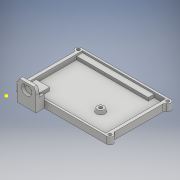
# Autodesk Inventor part: Redid DAQ Enclosure Bottom TTL
Saved by Autodesk Inventor 2017 (Build 210142000, 142)
## iProperties
Created: 2017-07-24
Part Number: Redid DAQ Enclosure Bottom TTL
Material: Generic
Document SubType Name: Modeling
Designer: andrew
Density: 1 g/cm^3
Appearance: Default
Author: andrew
Autodesk Inventor part; units mm, degrees
ref_plane "YZ Plane" through (0, 0, 0) normal (1, 0, 0) x (0, 1, 0)
ref_plane "XZ Plane" through (0, 0, 0) normal (0, 1, 0) x (-1, 0, 0)
ref_plane "XY Plane" through (0, 0, 0) normal (0, 0, 1) x (1, 0, 0)
sketch "Sketch1" plane through (0, 0, 0) normal (0, 0, 1) x (1, 0, 0)
  line L0 (85.72, 30.226) -> (85.72, 1.401) construction
  line L1 (85.72, 1.401) -> (45.72, 1.401) construction
  line L2 (85.72, 1.401) -> (5.72, 1.401) construction
  line L3 (5.72, 1.401) -> (5.72, 59.001) construction
  line L4 (5.72, 59.001) -> (85.72, 59.001) construction
  line L5 (85.72, 59.001) -> (85.72, 1.401) construction
  line L6 (61.99, 1.401) -> (61.99, 20.221) construction
  line L7 (61.99, 20.221) -> (85.72, 20.221) construction
  line L8 (61.99, 20.221) -> (58.44, 20.221) construction
  line L9 (61.99, 23.771) -> (61.99, 20.221) construction
  line L10 (60.215, 20.221) -> (61.99, 20.221) construction
  line L11 (61.99, 20.221) -> (61.99, 21.996) construction
  line L12 (61.99, 21.996) -> (60.215, 21.996) construction
  line L13 (60.215, 21.996) -> (60.215, 20.221) construction
  circle A0 centre (60.215, 21.996) radius 1.775 construction
  circle A1 centre (60.215, 21.996) radius 2.775 construction
  circle A2 centre (60.215, 21.996) radius 4.275 construction
  line L14 (5.72, 59.001) -> (74.72, 59.001) construction
  line L15 (74.72, 59.001) -> (74.72, 53.301) construction
  line L16 (74.72, 53.301) -> (5.72, 53.301) construction
  line L17 (5.72, 53.301) -> (5.72, 59.001) construction
  line L18 (5.72, 1.401) -> (18.72, 1.401) construction
  line L19 (18.72, 1.401) -> (18.72, 14.401) construction
  line L20 (18.72, 14.401) -> (5.72, 14.401) construction
  line L21 (5.72, 14.401) -> (5.72, 1.401) construction
  circle A3 centre (2.72, 58.001) radius 1.5
  line L22 (3.72, 61.001) -> (5.72, 61.001)
  line L23 (5.72, 61.001) -> (5.72, 59.001) construction
  line L24 (5.72, 61.001) -> (2.72, 61.001)
  line L25 (5.72, 55.001) -> (5.72, 61.001) construction
  line L26 (45.72, 1.9437) -> (45.72, 30.226) construction
  line L27 (45.72, 30.226) -> (85.72, 30.226) construction
  arc A4 (2.72, 61.001) -> (1.52, 55.2515) centre (2.72, 58.001) ccw
  circle A5 centre (2.72, 2.451) radius 1.5
  line L28 (3.72, -0.549) -> (5.72, -0.549)
  line L29 (5.72, -0.549) -> (2.72, -0.549)
  arc A6 (1.52, 5.2005) -> (2.72, -0.549) centre (2.72, 2.451) ccw
  circle A7 centre (88.72, 58.001) radius 1.5
  line L30 (85.72, 61.001) -> (88.72, 61.001)
  arc A8 (89.92, 55.2515) -> (88.72, 61.001) centre (88.72, 58.001) ccw
  line L31 (85.72, -0.549) -> (88.72, -0.549)
  circle A9 centre (88.72, 2.451) radius 1.5
  arc A10 (88.72, -0.549) -> (89.92, 5.2005) centre (88.72, 2.451) ccw
  line L32 (2.72, 53.4184) -> (2.72, 7.0336)
  line L33 (5.72, 61.001) -> (85.72, 61.001)
  line L34 (88.72, 53.4184) -> (88.72, 7.0336)
  line L35 (85.72, -0.549) -> (5.72, -0.549)
  arc A11 (2.72, 53.4184) -> (1.52, 55.2515) centre (0.72, 53.4184) ccw
  arc A12 (1.52, 5.2005) -> (2.72, 7.0336) centre (0.72, 7.0336) ccw
  arc A13 (88.72, 7.0336) -> (89.92, 5.2005) centre (90.72, 7.0336) ccw
  arc A14 (89.92, 55.2515) -> (88.72, 53.4184) centre (90.72, 53.4184) ccw
  point P0 (0, 0)
  point P1 (2.72, 55.001)
  point P2 (2.72, 5.451)
  point P3 (91.44, 0)
  point P4 (88.72, 55.001)
  point P5 (88.72, 5.451)
  dimension "d32" = 40
  dimension "d33" = 28.825
  dimension "d34" = 80
  dimension "d37" = 18.82
  dimension "d40" = 5.55
  dimension "d41" = 8.55
  dimension "d42" = 69
  dimension "d43" = 5.7
  dimension "d44" = 13
  dimension "d45" = 13
  dimension "d52" = 2
  dimension "d80" = 3
  constraints: 72 end point, 20 point on circle, 17 symmetric about line, 14 centre point, 9 parallel, 8 tangent, 7 perpendicular, 6 horizontal, 6 point on line, 3 coincident, 3 equal radius, 2 midpoint, 2 vertical, 1 horizontal alignment, 8 other
  measures "d32" distance of L0.end L1.end
  measures "d33" distance of L0.start L0.end
  measures "d34" distance of L3.end L4.end
  measures "d37" distance of L6.start L6.end
  measures "d40" diameter of A1
  measures "d41" diameter of A2
  measures "d42" distance of L15.end L16.end
  measures "d43" distance of L14.end L15.end
  measures "d44" distance of L20.end L19.end
  measures "d45" distance of L19.end L18.end
  measures "d52" radius of A11
  measures "d80" diameter of A3
extrude "Extrusion1" add sketch "Sketch1" along normal blind 2
sketch "Sketch2" plane through (0, 0, 2) normal (0, 0, 1) x (1, 0, 0)
  line L0 (85.72, 30.226) -> (85.72, 1.401)
  line L1 (5.72, 14.401) -> (5.72, 53.301)
  line L2 (74.72, 59.001) -> (85.72, 59.001)
  line L3 (85.72, 59.001) -> (85.72, 1.401)
  line L4 (61.815, 21.996) -> (60.215, 21.996)
  circle A0 centre (60.215, 21.996) radius 1.6
  circle A1 centre (60.215, 21.996) radius 2.775 construction
  circle A2 centre (60.215, 21.996) radius 4.275
  line L5 (45.72, 59.001) -> (74.72, 59.001)
  line L6 (74.72, 59.001) -> (74.72, 53.301)
  line L7 (74.72, 53.301) -> (5.72, 53.301)
  line L8 (5.72, 58.001) -> (5.72, 59.001)
  line L9 (5.72, 1.401) -> (18.72, 1.401)
  line L10 (18.72, 1.401) -> (18.72, 14.401)
  line L11 (18.72, 14.401) -> (5.72, 14.401)
  line L12 (5.72, 2.451) -> (5.72, 1.401)
  circle A3 centre (2.72, 58.001) radius 1.5
  line L13 (3.72, 61.001) -> (5.72, 61.001)
  line L14 (5.72, 61.001) -> (5.72, 59.001)
  line L15 (5.72, 61.001) -> (2.72, 61.001)
  line L16 (5.72, 59.001) -> (5.72, 61.001)
  arc A4 (2.72, 61.001) -> (1.52, 55.2515) centre (2.72, 58.001) ccw
  line L17 (3.72, -0.549) -> (5.72, -0.549)
  line L18 (5.72, -0.549) -> (2.72, -0.549)
  circle A5 centre (2.72, 2.451) radius 1.5
  arc A6 (1.52, 5.2005) -> (2.72, -0.549) centre (2.72, 2.451) ccw
  line L19 (85.72, -0.549) -> (88.72, -0.549)
  circle A7 centre (88.72, 2.451) radius 1.5
  arc A8 (88.72, -0.549) -> (89.92, 5.2005) centre (88.72, 2.451) ccw
  circle A9 centre (88.72, 58.001) radius 1.5
  arc A10 (89.92, 55.2515) -> (88.72, 61.001) centre (88.72, 58.001) ccw
  line L20 (85.72, 61.001) -> (88.72, 61.001)
  line L21 (2.72, 53.4184) -> (2.72, 7.0336)
  line L22 (5.72, 61.001) -> (85.72, 61.001)
  line L23 (88.72, 53.4184) -> (88.72, 7.0336)
  line L24 (85.72, -0.549) -> (5.72, -0.549)
  arc A11 (2.72, 53.4184) -> (1.52, 55.2515) centre (0.72, 53.4184) ccw
  arc A12 (1.52, 5.2005) -> (2.72, 7.0336) centre (0.72, 7.0336) ccw
  arc A13 (88.72, 7.0336) -> (89.92, 5.2005) centre (90.72, 7.0336) ccw
  arc A14 (89.92, 55.2515) -> (88.72, 53.4184) centre (90.72, 53.4184) ccw
  line L25 (85.72, 1.401) -> (74.72, 1.401)
  line L26 (61.99, 1.401) -> (45.72, 1.401)
  line L27 (85.72, 1.401) -> (74.72, 1.401)
  line L28 (61.99, 1.401) -> (18.72, 1.401)
  line L29 (61.99, 1.401) -> (74.72, 1.401)
  point P0 (0, 0)
  point P1 (2.72, 55.001)
  point P2 (2.72, 5.451)
  point P3 (91.44, 0)
  point P4 (88.72, 5.451)
  point P5 (88.72, 55.001)
  dimension "d89" = 3.2
  dimension "d53" = 40
  dimension "d54" = 28.825
  dimension "d55" = 80
  dimension "d57" = 5.55
  dimension "d58" = 8.55
  dimension "d59" = 69
  dimension "d60" = 5.7
  dimension "d61" = 13
  dimension "d62" = 13
  dimension "d63" = 2
  dimension "d81" = 3
  dimension "d82" = 3
  dimension "d83" = 3
  dimension "d84" = 3
  constraints: 60 end point, 22 point on circle, 14 centre point, 8 parallel, 8 tangent, 6 horizontal, 5 perpendicular, 5 point on line, 3 coincident, 3 equal radius, 1 horizontal alignment, 1 vertical, 2 other
  measures "d53" distance of L0.end L26.end
  measures "d54" distance of L0.start L0.end
  measures "d55" distance of L8.end L3.start
  measures "d57" diameter of A1
  measures "d58" diameter of A2
  measures "d59" distance of L7.end L6.end
  measures "d60" distance of L6.start L6.end
  measures "d61" distance of L1.start L11.start
  measures "d62" distance of L9.end L11.start
  measures "d63" radius of A11
  measures "d81" diameter of A3
  measures "d82" diameter of A5
  measures "d83" diameter of A7
  measures "d84" diameter of A9
extrude "Extrusion2" add sketch "Sketch2" along normal blind 3
sketch "Sketch5" plane through (0, 0, 5) normal (0, 0, 1) x (1, 0, 0)
  line L0 (85.72, 30.226) -> (85.72, 1.401)
  line L1 (85.72, 1.401) -> (45.72, 1.401)
  line L2 (85.72, 1.401) -> (5.72, 1.401)
  line L3 (5.72, 1.401) -> (5.72, 59.001)
  line L4 (5.72, 59.001) -> (85.72, 59.001)
  line L5 (85.72, 59.001) -> (85.72, 1.401)
  line L6 (5.72, 59.001) -> (74.72, 59.001)
  line L7 (5.72, 53.301) -> (5.72, 59.001)
  line L8 (5.72, 1.401) -> (18.72, 1.401)
  line L9 (5.72, 14.401) -> (5.72, 1.401)
  circle A0 centre (2.72, 58.001) radius 1.5
  line L10 (3.72, 61.001) -> (5.72, 61.001)
  line L11 (5.72, 61.001) -> (5.72, 59.001)
  line L12 (5.72, 61.001) -> (2.72, 61.001)
  line L13 (5.72, 55.001) -> (5.72, 61.001)
  arc A1 (2.72, 61.001) -> (1.52, 55.2515) centre (2.72, 58.001) ccw
  line L14 (3.72, -0.549) -> (5.72, -0.549)
  line L15 (5.72, -0.549) -> (2.72, -0.549)
  circle A2 centre (2.72, 2.451) radius 1.5
  arc A3 (1.52, 5.2005) -> (2.72, -0.549) centre (2.72, 2.451) ccw
  line L16 (85.72, -0.549) -> (88.72, -0.549)
  circle A4 centre (88.72, 2.451) radius 1.5
  arc A5 (88.72, -0.549) -> (89.92, 5.2005) centre (88.72, 2.451) ccw
  circle A6 centre (88.72, 58.001) radius 1.5
  arc A7 (89.92, 55.2515) -> (88.72, 61.001) centre (88.72, 58.001) ccw
  line L17 (85.72, 61.001) -> (88.72, 61.001)
  line L18 (2.72, 53.4184) -> (2.72, 7.0336)
  line L19 (5.72, 61.001) -> (85.72, 61.001)
  line L20 (88.72, 53.4184) -> (88.72, 7.0336)
  line L21 (85.72, -0.549) -> (5.72, -0.549)
  arc A8 (2.72, 53.4184) -> (1.52, 55.2515) centre (0.72, 53.4184) ccw
  arc A9 (1.52, 5.2005) -> (2.72, 7.0336) centre (0.72, 7.0336) ccw
  arc A10 (88.72, 7.0336) -> (89.92, 5.2005) centre (90.72, 7.0336) ccw
  arc A11 (89.92, 55.2515) -> (88.72, 53.4184) centre (90.72, 53.4184) ccw
  point P0 (0, 0)
  point P1 (0, 0)
  point P2 (2.72, 55.001)
  point P3 (2.72, 5.451)
  point P4 (91.44, 0)
  point P5 (88.72, 5.451)
  point P6 (88.72, 55.001)
  dimension "d64" = 40
  dimension "d65" = 28.825
  dimension "d66" = 80
  dimension "d74" = 2
  dimension "d85" = 3
  dimension "d86" = 3
  dimension "d87" = 3
  dimension "d88" = 3
  constraints: 44 end point, 20 point on circle, 12 centre point, 8 tangent, 4 horizontal, 4 point on line, 3 equal radius, 3 parallel, 2 perpendicular, 1 vertical
  measures "d64" distance of L0.end L1.end
  measures "d65" distance of L0.start L0.end
  measures "d66" distance of L6.start L4.end
  measures "d74" radius of A8
  measures "d85" diameter of A0
  measures "d86" diameter of A2
  measures "d87" diameter of A4
  measures "d88" diameter of A6
extrude "Extrusion5" add sketch "Sketch5" along normal blind 1.67
chamfer "Chamfer1" distance 1 distance2 3 1 edges at (55.94, 21.996, 5) measured on face at (63.5414, 21.5273, 5)
sketch "Sketch6" plane through (2.72, -0.549, 0) normal (0, -1, 0) x (1, 0, 0)
  line L0 (-2.72, 20.7114) -> (-2.72, 7.1986) construction
  arc A0 (14.6348, 17.447) -> (18.9452, 17.447) centre (16.79, 14.78) ccw construction
  line L1 (14.6347, 17.447) -> (18.9453, 17.447) construction
  line L2 (-3, 20.67) -> (-3, 6.67) construction
  line L3 (0, 13.555) -> (92, 13.555) construction
  line L4 (0.28, 13.555) -> (46, 13.555) construction
  line L5 (13.7208, 18.67) -> (19.8592, 18.67)
  line L6 (8.6741, 18.67) -> (83, 18.67) construction
  line L7 (83, 18.67) -> (8.6741, 18.67) construction
  circle A1 centre (16.79, 14.78) radius 7.15 construction
  circle A2 centre (16.79, 14.78) radius 6.25 construction
  line L8 (18.077, 2.0446) -> (21.077, 2.0446)
  line L9 (13.0545, 18.0609) -> (13.0545, 18.67) construction
  line L10 (11.835, 14.78) -> (11.4131, 5.117) construction
  line L11 (11.835, 14.78) -> (21.5072, 14.78) construction
  line L12 (21.745, 14.78) -> (22.1562, 5.3611) construction
  line L13 (21.745, 14.78) -> (31.1729, 14.78) construction
  arc A3 (13.7208, 18.67) -> (21.5912, 13.555) centre (16.79, 14.78) ccw
  arc A4 (21.5912, 13.555) -> (19.8592, 18.67) centre (16.79, 14.78) ccw
  line L14 (22.1562, 5.3611) -> (11.4131, 5.117) construction
  line L15 (-3, 20.67) -> (-3, 6.67)
  line L16 (0, 6.67) -> (-3, 6.67) projected
  arc A5 (9.985, 20.67) -> (23.595, 20.67) centre (16.79, 14.78) ccw
  line L17 (16.79, 14.78) -> (7.79, 14.78) construction
  line L18 (7.79, 14.78) -> (7.79, 0)
  line L19 (86, 0) -> (0, 0) projected
  line L20 (16.79, 14.78) -> (25.79, 14.78) construction
  line L21 (25.79, 14.78) -> (25.79, 0)
  line L22 (-3, 20.67) -> (-2.72, 20.67)
  line L23 (9.985, 20.67) -> (35.5259, 20.67)
  point P0 (-2.72, 0)
  point P1 (-2.72, 20.67)
  point P2 (-1.2, 6.67)
  dimension "d90" = 14.3
  dimension "d91" = 12.5
  dimension "d92" = 3
  dimension "d93" = 92.5
  dimension "d94" = 87.5
  constraints: 44 end point, 13 point on circle, 9 point on line, 6 centre point, 6 horizontal, 3 coincident, 3 perpendicular, 2 equal length
  measures "d90" diameter of A1
  measures "d91" diameter of A2
  measures "d92" distance of L8.start L8.end
  measures "d93" angle of L10 L11
  measures "d94" angle of L12 L13
extrude "Extrusion6" add sketch "Sketch6" along normal blind 8
sketch "Sketch7" plane through (2.72, -8.549, 0) normal (0, -1, 0) x (1, 0, 0)
  point P0 (-2.72, 0)
sketch "Sketch8" plane through (2.72, -0.549, 0) normal (0, 1, 0) x (1, 0, 0)
  line L0 (18.077, 2.0446) -> (21.077, 2.0446)
  line L1 (86, 0) -> (0, 0) construction
  line L2 (22.1562, -5.3611) -> (11.4131, -5.117) construction
  line L3 (18.077, -2.0446) -> (21.077, -2.0446) construction
  line L4 (-2.72, -20.7114) -> (-2.72, -7.1986) construction
  line L5 (-3, -20.67) -> (-3, -6.67) construction
  line L6 (-3, -20.67) -> (-3, -6.67)
  line L7 (0, -13.555) -> (92, -13.555) construction
  line L8 (0.28, -13.555) -> (46, -13.555) construction
  line L9 (0, -6.67) -> (-3, -6.67)
  line L10 (7.79, -14.78) -> (7.79, 0) construction
  line L11 (25.79, -14.78) -> (25.79, 0) construction
  line L12 (-3, -20.67) -> (-2.72, -20.67)
  line L13 (13.04, -8.2848) -> (20.54, -8.2848) construction
  line L14 (20.54, -8.2848) -> (24.29, -14.78) construction
  line L15 (22.415, -11.5324) -> (28.3907, -11.5324) construction
  line L16 (27.6858, -27.8063) -> (6.6122, -26.5118)
  line L17 (6.6122, -26.5118) -> (5.8176, -11.5324)
  arc A0 (21.5912, -13.555) -> (20.5323, -11.5324) centre (16.79, -14.78) ccw construction
  line L18 (28.3907, -11.5324) -> (23.5504, -11.5324)
  line L19 (10.0296, -11.5324) -> (5.8176, -11.5324)
  arc A1 (23.5504, -11.5324) -> (10.0296, -11.5324) centre (16.79, -14.78) ccw
  line L20 (28.3907, -11.5324) -> (27.6858, -27.8063)
  point P0 (-2.72, 0)
  point P1 (-2.72, 0)
  point P2 (-2.72, -20.67)
  point P3 (-1.2, -6.67)
  constraints: 42 end point, 4 point on circle, 4 point on line, 2 centre point, 2 horizontal, 2 midpoint, 2 symmetric about line
extrude "Extrusion7" cut sketch "Sketch8" against normal blind 5
body "Solid1"
